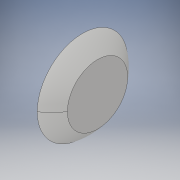
# Autodesk Inventor part: Leaf
Saved by Autodesk Inventor 2019 (Build 230136000, 136)
## iProperties
Created: 2019-11-16
Part Number: Leaf
Material: Generic
Document SubType Name: Modeling
Designer: Jorian Brusind
Density: 1 g/cm^3
Appearance: Default
Author: Jorian Brusind
Autodesk Inventor part; units mm, degrees
ref_plane "YZ Plane" through (0, 0, 0) normal (1, 0, 0) x (0, 1, 0)
ref_plane "XZ Plane" through (0, 0, 0) normal (0, 1, 0) x (-1, 0, 0)
ref_plane "XY Plane" through (0, 0, 0) normal (0, 0, 1) x (1, 0, 0)
sketch "Sketch1" plane through (0, 0, 0) normal (0, 1, 0) x (-1, 0, 0)
  line L0 (0, 0) -> (-10, 0)
  line L1 (-10, 0) -> (-10, -20)
  line L2 (-10, 0) -> (-10, 20)
  line L3 (0, 0) -> (0, 30)
  line L4 (0, 0) -> (0, -30)
  spline S0 degree 2 poles (0, 30) (-4.6494, 26.8211) (-10, 20) knots 0 0 0 1 1 1
  spline S1 degree 2 poles (0, -30) (-4.6494, -26.8211) (-10, -20) knots 0 0 0 1 1 1
  point P0 (-4.2835, 26.4431)
  point P1 (-4.2835, -26.4431)
  dimension "d0" = 10
  dimension "d1" = 20
  dimension "d2" = 20
  dimension "d3" = 30
  dimension "d4" = 30
  constraints: 10 end point, 3 vertical, 1 horizontal, 1 perpendicular, 1 symmetric about line, 6 other
  measures "d0" distance of L0.start L0.end
  measures "d1" distance of L0.end L1.end
  measures "d2" distance of L0.end L2.end
  measures "d3" distance of L0.start L3.end
  measures "d4" distance of L0.start L4.end
revolve "Revolution1" add sketch "Sketch1" angle 360 about axis through (0, 0, 0) along (1, 0, 0) contours L0 L2 S0 L3
shell "Shell1" thickness 3 removed faces 1 at (0, 4.6472, -8.8546)
body "Solid1"
